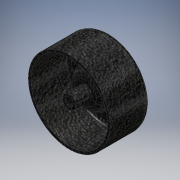
# Autodesk Inventor part: kolo
Saved by Autodesk Inventor 2018 (Build 220112000, 112)
## iProperties
Created: 2023-12-05
Part Number: kolo
Material: Všeobecné
Document SubType Name: Modeling
Designer: 42073
Density: 1 g/cm^3
Appearance: Černý – litý
Author: 42073
Autodesk Inventor part; units mm, degrees
ref_plane "YZ Plane" through (0, 0, 0) normal (1, 0, 0) x (0, 1, 0)
ref_plane "XY Plane" through (0, 0, 0) normal (0, 0, 1) x (1, 0, 0)
sketch "Náčrt1" plane through (0, 0, 0) normal (0, 0, 1) x (1, 0, 0)
  line L0 (0, 0) -> (0, 14.75)
  line L1 (0, 0) -> (15, 0)
  line L2 (15, 0) -> (15, 7)
  line L3 (15, 7) -> (9, 7)
  line L4 (9, 7) -> (9, 14.75)
  arc A0 (9, 14.75) -> (0, 14.75) centre (4.5, -25.625) ccw
  dimension "d1" = 15
  dimension "d2" = 7
  dimension "d3" = 6
  constraints: 10 end point, 3 perpendicular, 2 point on circle, 1 centre point, 1 horizontal, 1 vertical
  measures "d1" distance of L0.start L1.end
  measures "d2" distance of L1.end L2.end
  measures "d3" distance of L2.end L3.end
revolve "Rotace1" add sketch "Náčrt1" angle 360 about axis through (15, 0, 0) along (0, 1, 0)
sketch "Náčrt2" plane through (15, 0, 0) normal (0, -1, 0) x (1, 0, 0)
  circle A0 centre (0, 0) radius 1.5
  point P0 (-15, 0)
  dimension "d6" = 3
  constraints: 1 centre point
  measures "d6" diameter of A0
extrude "Vysunutí1" cut sketch "Náčrt2" against normal blind 10
fillet "Zaoblení1" radius 2 3 edges at (21, 7, 0) (21, 14.75, 0) (30, 14.75, 0)
shell "Skořepina1" thickness 1 removed faces 1 at (4.6453, 0, -1.1966)
ref_plane "Pracovní rovina1" through (0, 15.25, 0) normal (0, 1, 0) x (-1, 0, 0)
sketch "Náčrt3" plane through (0, 15.25, 0) normal (0, 1, 0) x (-1, 0, 0)
  circle A0 centre (-15, 0) radius 1.5 projected
  circle A1 centre (-15, 0) radius 9.5
  line L0 (-24.5881, -0.0196) -> (-27.472, 1.4048)
  line L1 (-27.472, 1.4048) -> (-27.4055, 1.8993)
  line L2 (-27.4055, 1.8993) -> (-24.2478, 2.5116)
  line L3 (-24.2478, 2.5116) -> (-24.3048, 2.0881)
  line L4 (-24.3048, 2.0881) -> (-25.1862, 1.9275)
  line L5 (-25.1862, 1.9275) -> (-25.3412, 0.7745)
  line L6 (-25.3412, 0.7745) -> (-24.5335, 0.3868)
  line L7 (-24.5335, 0.3868) -> (-24.5881, -0.0196)
  line L8 (-25.5437, 1.8634) -> (-27.0288, 1.587)
  line L9 (-27.0288, 1.587) -> (-25.6691, 0.9307)
  line L10 (-25.6691, 0.9307) -> (-25.5437, 1.8634)
  line L11 (-23.4586, 4.4131) -> (-23.6046, 4.0565)
  line L12 (-23.6046, 4.0565) -> (-23.8195, 4.1445)
  spline S0 degree 2 poles (-23.8195, 4.1445) (-23.7846, 4.0341) (-23.7427, 3.8755) (-23.7376, 3.7773) knots 0 0 0 1 2 2 2
  spline S1 degree 2 poles (-23.7376, 3.7773) (-23.7319, 3.6869) (-23.7595, 3.5087) (-23.8034, 3.4013) knots 0 0 0 1 2 2 2
  spline S2 degree 2 poles (-23.8034, 3.4013) (-23.8746, 3.2275) (-24.1384, 2.9939) (-24.3199, 2.9481) knots 0 0 0 1 2 2 2
  spline S3 degree 2 poles (-24.3199, 2.9481) (-24.5015, 2.9023) (-24.9597, 2.9565) (-25.2272, 3.066) knots 0 0 0 1 2 2 2
  spline S4 degree 2 poles (-25.2272, 3.066) (-25.506, 3.1802) (-25.854, 3.4908) (-25.9556, 3.6792) knots 0 0 0 1 2 2 2
  spline S5 degree 2 poles (-25.9556, 3.6792) (-26.0451, 3.8519) (-26.069, 4.2434) (-25.995, 4.4239) knots 0 0 0 1 2 2 2
  spline S6 degree 2 poles (-25.995, 4.4239) (-25.9305, 4.5817) (-25.7632, 4.7881) (-25.6367, 4.8885) knots 0 0 0 1 2 2 2
  line L13 (-25.6367, 4.8885) -> (-26.5511, 5.2628)
  line L14 (-26.5511, 5.2628) -> (-26.4051, 5.6194)
  line L15 (-26.4051, 5.6194) -> (-23.4586, 4.4131)
  line L16 (-24.1189, 4.2671) -> (-25.3418, 4.7677)
  spline S7 degree 2 poles (-25.3418, 4.7677) (-25.4601, 4.6614) (-25.5942, 4.4707) (-25.6438, 4.3496) knots 0 0 0 1 2 2 2
  spline S8 degree 2 poles (-25.6438, 4.3496) (-25.7561, 4.0752) (-25.4719, 3.5959) (-25.0833, 3.4368) knots 0 0 0 1 2 2 2
  spline S9 degree 2 poles (-25.0833, 3.4368) (-24.7085, 3.2834) (-24.2157, 3.3592) (-24.1081, 3.6221) knots 0 0 0 1 2 2 2
  spline S10 degree 2 poles (-24.1081, 3.6221) (-24.051, 3.7615) (-24.0629, 4.0974) (-24.1189, 4.2671) knots 0 0 0 1 2 2 2
  spline S11 degree 2 poles (-22.5603, 5.669) (-22.8813, 5.2245) (-23.7328, 5.096) (-24.1933, 5.4287) knots 0 0 0 1 2 2 2
  spline S12 degree 2 poles (-24.1933, 5.4287) (-24.6459, 5.7555) (-24.8398, 6.6176) (-24.5635, 7.0001) knots 0 0 0 1 2 2 2
  spline S13 degree 2 poles (-24.5635, 7.0001) (-24.4392, 7.1723) (-24.1467, 7.3663) (-23.9697, 7.3878) knots 0 0 0 1 2 2 2
  spline S14 degree 2 poles (-23.9697, 7.3878) (-23.7913, 7.4112) (-23.4083, 7.2961) (-23.186, 7.1356) knots 0 0 0 1 2 2 2
  line L17 (-23.186, 7.1356) -> (-23.0158, 7.0127)
  line L18 (-23.0158, 7.0127) -> (-23.9428, 5.7291)
  spline S15 degree 2 poles (-23.9428, 5.7291) (-23.6204, 5.4963) (-23.0437, 5.5734) (-22.8355, 5.8617) knots 0 0 0 1 2 2 2
  spline S16 degree 2 poles (-22.8355, 5.8617) (-22.7617, 5.9638) (-22.6646, 6.1953) (-22.6428, 6.3015) knots 0 0 0 1 2 2 2
  spline S17 degree 2 poles (-22.6428, 6.3015) (-22.6221, 6.4145) (-22.6083, 6.5812) (-22.6129, 6.6424) knots 0 0 0 1 2 2 2
  line L19 (-22.6129, 6.6424) -> (-22.5999, 6.6604)
  line L20 (-22.5999, 6.6604) -> (-22.2595, 6.4146)
  spline S18 degree 2 poles (-22.2595, 6.4146) (-22.2765, 6.3446) (-22.331, 6.1342) (-22.3593, 6.0571) knots 0 0 0 1 2 2 2
  spline S19 degree 2 poles (-22.3593, 6.0571) (-22.3983, 5.9482) (-22.4793, 5.7812) (-22.5603, 5.669) knots 0 0 0 1 2 2 2
  spline S20 degree 2 poles (-23.4739, 6.8804) (-23.6029, 6.9675) (-23.8248, 7.0485) (-23.923, 7.0433) knots 0 0 0 1 2 2 2
  spline S21 degree 2 poles (-23.923, 7.0433) (-24.0321, 7.0398) (-24.2291, 6.9231) (-24.3203, 6.797) knots 0 0 0 1 2 2 2
  spline S22 degree 2 poles (-24.3203, 6.797) (-24.4099, 6.6728) (-24.4616, 6.4451) (-24.4416, 6.321) knots 0 0 0 1 2 2 2
  spline S23 degree 2 poles (-24.4416, 6.321) (-24.4182, 6.1974) (-24.292, 5.9966) (-24.1811, 5.9012) knots 0 0 0 1 2 2 2
  line L21 (-24.1811, 5.9012) -> (-23.4739, 6.8804)
  spline S24 degree 2 poles (-21.1682, 8.734) (-20.7912, 8.2959) (-20.8017, 7.456) (-21.1536, 7.1531) knots 0 0 0 1 2 2 2
  spline S25 degree 2 poles (-21.1536, 7.1531) (-21.515, 6.8421) (-22.3525, 6.9785) (-22.7166, 7.4016) knots 0 0 0 1 2 2 2
  spline S26 degree 2 poles (-22.7166, 7.4016) (-23.0904, 7.836) (-23.0775, 8.6845) (-22.7293, 8.9841) knots 0 0 0 1 2 2 2
  spline S27 degree 2 poles (-22.7293, 8.9841) (-22.3773, 9.287) (-21.5436, 9.1702) (-21.1682, 8.734) knots 0 0 0 1 2 2 2
  spline S28 degree 2 poles (-21.4697, 8.4746) (-21.7597, 8.8116) (-22.2869, 8.9282) (-22.5134, 8.7333) knots 0 0 0 1 2 2 2
  spline S29 degree 2 poles (-22.5134, 8.7333) (-22.74, 8.5383) (-22.7052, 7.998) (-22.4152, 7.661) knots 0 0 0 1 2 2 2
  spline S30 degree 2 poles (-22.4152, 7.661) (-22.1332, 7.3334) (-21.5961, 7.209) (-21.3695, 7.404) knots 0 0 0 1 2 2 2
  spline S31 degree 2 poles (-21.3695, 7.404) (-21.1449, 7.5973) (-21.1829, 8.1413) (-21.4697, 8.4746) knots 0 0 0 1 2 2 2
  line L22 (-18.4856, 8.8838) -> (-18.8293, 8.7096)
  line L23 (-18.8293, 8.7096) -> (-19.4189, 9.873)
  spline S32 degree 2 poles (-19.4189, 9.873) (-19.4903, 10.014) (-19.6396, 10.2429) (-19.7161, 10.2955) knots 0 0 0 1 2 2 2
  spline S33 degree 2 poles (-19.7161, 10.2955) (-19.797, 10.3514) (-19.9848, 10.3504) (-20.1126, 10.2857) knots 0 0 0 1 2 2 2
  spline S34 degree 2 poles (-20.1126, 10.2857) (-20.2404, 10.2209) (-20.4421, 9.947) (-20.5163, 9.771) knots 0 0 0 1 2 2 2
  line L24 (-20.5163, 9.771) -> (-19.7437, 8.2463)
  line L25 (-19.7437, 8.2463) -> (-20.0874, 8.0721)
  line L26 (-20.0874, 8.0721) -> (-21.1213, 10.1123)
  line L27 (-21.1213, 10.1123) -> (-20.7776, 10.2865)
  line L28 (-20.7776, 10.2865) -> (-20.6626, 10.0596)
  spline S35 degree 2 poles (-20.6626, 10.0596) (-20.5787, 10.2765) (-20.3549, 10.5727) (-20.1875, 10.6575) knots 0 0 0 1 2 2 2
  spline S36 degree 2 poles (-20.1875, 10.6575) (-19.8878, 10.8094) (-19.3476, 10.5847) (-19.1566, 10.208) knots 0 0 0 1 2 2 2
  line L29 (-19.1566, 10.208) -> (-18.4856, 8.8838)
  line L30 (-15.1164, 12.231) -> (-16.5279, 12.0972)
  line L31 (-16.5279, 12.0972) -> (-16.4467, 11.2414)
  line L32 (-16.4467, 11.2414) -> (-15.0943, 11.3697)
  line L33 (-15.0943, 11.3697) -> (-15.0603, 11.0107)
  line L34 (-15.0603, 11.0107) -> (-16.4127, 10.8824)
  line L35 (-16.4127, 10.8824) -> (-16.2742, 9.4218)
  line L36 (-16.2742, 9.4218) -> (-16.6775, 9.3836)
  line L37 (-16.6775, 9.3836) -> (-16.9652, 12.4179)
  line L38 (-16.9652, 12.4179) -> (-15.1505, 12.59)
  line L39 (-15.1505, 12.59) -> (-15.1164, 12.231)
  line L40 (-12.8787, 9.2951) -> (-14.3511, 9.5023)
  line L41 (-14.3511, 9.5023) -> (-14.3078, 9.8105)
  line L42 (-14.3078, 9.8105) -> (-13.7599, 9.7334)
  line L43 (-13.7599, 9.7334) -> (-13.4752, 11.7562)
  line L44 (-13.4752, 11.7562) -> (-14.0231, 11.8333)
  line L45 (-14.0231, 11.8333) -> (-13.9842, 12.1096)
  spline S37 degree 2 poles (-13.9842, 12.1096) (-13.6736, 12.0659) (-13.3553, 12.2007) (-13.3013, 12.4426) knots 0 0 0 1 2 2 2
  line L46 (-13.3013, 12.4426) -> (-12.9882, 12.3985)
  line L47 (-12.9882, 12.3985) -> (-13.371, 9.6786)
  line L48 (-13.371, 9.6786) -> (-12.8353, 9.6033)
  line L49 (-12.8353, 9.6033) -> (-12.8787, 9.2951)
  line L50 (-10.4121, 8.3212) -> (-9.0641, 10.6461)
  line L51 (-9.0641, 10.6461) -> (-9.9487, 11.159)
  line L52 (-9.9487, 11.159) -> (-9.7678, 11.471)
  line L53 (-9.7678, 11.471) -> (-7.6481, 10.2419)
  line L54 (-7.6481, 10.2419) -> (-7.829, 9.9299)
  line L55 (-7.829, 9.9299) -> (-8.7136, 10.4429)
  line L56 (-8.7136, 10.4429) -> (-10.0616, 8.118)
  line L57 (-10.0616, 8.118) -> (-10.4121, 8.3212)
  spline S38 degree 2 poles (-8.3061, 6.6699) (-8.7001, 7.0514) (-8.7052, 7.9125) (-8.31, 8.3206) knots 0 0 0 1 2 2 2
  spline S39 degree 2 poles (-8.31, 8.3206) (-7.9217, 8.7216) (-7.0407, 8.79) (-6.7018, 8.4618) knots 0 0 0 1 2 2 2
  spline S40 degree 2 poles (-6.7018, 8.4618) (-6.5492, 8.314) (-6.3991, 7.9968) (-6.4032, 7.8185) knots 0 0 0 1 2 2 2
  spline S41 degree 2 poles (-6.4032, 7.8185) (-6.4055, 7.6386) (-6.5744, 7.276) (-6.7651, 7.0791) knots 0 0 0 1 2 2 2
  line L58 (-6.7651, 7.0791) -> (-6.9111, 6.9282)
  line L59 (-6.9111, 6.9282) -> (-8.0486, 8.0296)
  spline S42 degree 2 poles (-8.0486, 8.0296) (-8.3252, 7.7439) (-8.3315, 7.1621) (-8.076, 6.9147) knots 0 0 0 1 2 2 2
  spline S43 degree 2 poles (-8.076, 6.9147) (-7.9855, 6.8271) (-7.7703, 6.6978) (-7.6684, 6.661) knots 0 0 0 1 2 2 2
  spline S44 degree 2 poles (-7.6684, 6.661) (-7.5595, 6.6243) (-7.3965, 6.5868) (-7.3353, 6.5825) knots 0 0 0 1 2 2 2
  line L60 (-7.3353, 6.5825) -> (-7.3193, 6.5671)
  line L61 (-7.3193, 6.5671) -> (-7.6114, 6.2654)
  spline S45 degree 2 poles (-7.6114, 6.2654) (-7.6782, 6.2923) (-7.8787, 6.3764) (-7.9509, 6.4154) knots 0 0 0 1 2 2 2
  spline S46 degree 2 poles (-7.9509, 6.4154) (-8.0531, 6.4696) (-8.2068, 6.5737) (-8.3061, 6.6699) knots 0 0 0 1 2 2 2
  spline S47 degree 2 poles (-6.9764, 7.4006) (-6.8717, 7.5158) (-6.7597, 7.7237) (-6.7508, 7.8217) knots 0 0 0 1 2 2 2
  spline S48 degree 2 poles (-6.7508, 7.8217) (-6.7386, 7.9302) (-6.8259, 8.1419) (-6.9377, 8.2501) knots 0 0 0 1 2 2 2
  spline S49 degree 2 poles (-6.9377, 8.2501) (-7.0477, 8.3567) (-7.2656, 8.4405) (-7.3914, 8.4385) knots 0 0 0 1 2 2 2
  spline S50 degree 2 poles (-7.3914, 8.4385) (-7.5171, 8.4329) (-7.7339, 8.3369) (-7.8441, 8.2408) knots 0 0 0 1 2 2 2
  line L62 (-7.8441, 8.2408) -> (-6.9764, 7.4006)
  spline S51 degree 2 poles (-6.5566, 4.8808) (-6.6111, 4.9016) (-6.8004, 4.9679) (-6.8716, 5.0103) knots 0 0 0 1 2 2 2
  spline S52 degree 2 poles (-6.8716, 5.0103) (-6.972, 5.0662) (-7.1226, 5.1955) (-7.216, 5.341) knots 0 0 0 1 2 2 2
  spline S53 degree 2 poles (-7.216, 5.341) (-7.292, 5.4595) (-7.34, 5.731) (-7.311, 5.8641) knots 0 0 0 1 2 2 2
  spline S54 degree 2 poles (-7.311, 5.8641) (-7.2814, 5.9917) (-7.1086, 6.2347) (-6.9797, 6.3174) knots 0 0 0 1 2 2 2
  spline S55 degree 2 poles (-6.9797, 6.3174) (-6.7802, 6.4455) (-6.3894, 6.4586) (-6.1909, 6.3277) knots 0 0 0 1 2 2 2
  spline S56 degree 2 poles (-6.1909, 6.3277) (-6.012, 6.2136) (-5.6731, 5.8089) (-5.4944, 5.5626) knots 0 0 0 1 2 2 2
  line L63 (-5.4944, 5.5626) -> (-5.432, 5.6026)
  spline S57 degree 2 poles (-5.432, 5.6026) (-5.3198, 5.6746) (-5.2245, 5.8326) (-5.2251, 5.9203) knots 0 0 0 1 2 2 2
  spline S58 degree 2 poles (-5.2251, 5.9203) (-5.2256, 6.0081) (-5.3154, 6.2028) (-5.3768, 6.2985) knots 0 0 0 1 2 2 2
  spline S59 degree 2 poles (-5.3768, 6.2985) (-5.4488, 6.4107) (-5.7101, 6.6715) (-5.872, 6.7819) knots 0 0 0 1 2 2 2
  line L64 (-5.872, 6.7819) -> (-5.884, 6.8006)
  line L65 (-5.884, 6.8006) -> (-5.5535, 7.0127)
  spline S60 degree 2 poles (-5.5535, 7.0127) (-5.4712, 6.9393) (-5.194, 6.6447) (-5.0886, 6.4805) knots 0 0 0 1 2 2 2
  spline S61 degree 2 poles (-5.0886, 6.4805) (-4.9605, 6.2809) (-4.8481, 5.9686) (-4.8598, 5.8085) knots 0 0 0 1 2 2 2
  spline S62 degree 2 poles (-4.8598, 5.8085) (-4.8707, 5.6518) (-5.0555, 5.3864) (-5.2364, 5.2703) knots 0 0 0 1 2 2 2
  line L66 (-5.2364, 5.2703) -> (-6.5522, 4.4258)
  line L67 (-6.5522, 4.4258) -> (-6.7603, 4.7501)
  line L68 (-6.7603, 4.7501) -> (-6.5566, 4.8808)
  line L69 (-6.2864, 5.0542) -> (-5.7522, 5.3971)
  spline S63 degree 2 poles (-5.7522, 5.3971) (-5.8373, 5.5069) (-6.0981, 5.8355) (-6.2021, 5.9243) knots 0 0 0 1 2 2 2
  spline S64 degree 2 poles (-6.2021, 5.9243) (-6.3243, 6.0278) (-6.5966, 6.0908) (-6.7421, 5.9974) knots 0 0 0 1 2 2 2
  spline S65 degree 2 poles (-6.7421, 5.9974) (-6.9084, 5.8907) (-6.9566, 5.5955) (-6.8419, 5.4168) knots 0 0 0 1 2 2 2
  spline S66 degree 2 poles (-6.8419, 5.4168) (-6.7445, 5.265) (-6.4535, 5.0996) (-6.2864, 5.0542) knots 0 0 0 1 2 2 2
  line L70 (-5.5505, 1.4817) -> (-4.2753, 1.8375)
  spline S67 degree 2 poles (-4.2753, 1.8375) (-4.123, 1.88) (-3.8704, 1.9762) (-3.8096, 2.0341) knots 0 0 0 1 2 2 2
  spline S68 degree 2 poles (-3.8096, 2.0341) (-3.7417, 2.0941) (-3.7061, 2.2605) (-3.7413, 2.3866) knots 0 0 0 1 2 2 2
  spline S69 degree 2 poles (-3.7413, 2.3866) (-3.7731, 2.5008) (-3.9865, 2.7233) (-4.1583, 2.8241) knots 0 0 0 1 2 2 2
  spline S70 degree 2 poles (-4.1583, 2.8241) (-4.1909, 2.8125) (-4.2824, 2.7818) (-4.3442, 2.7645) knots 0 0 0 1 2 2 2
  line L71 (-4.3442, 2.7645) -> (-5.7955, 2.3596)
  line L72 (-5.7955, 2.3596) -> (-5.8991, 2.7307)
  line L73 (-5.8991, 2.7307) -> (-4.6239, 3.0866)
  spline S71 degree 2 poles (-4.6239, 3.0866) (-4.4716, 3.129) (-4.2189, 3.2252) (-4.1582, 3.2832) knots 0 0 0 1 2 2 2
  spline S72 degree 2 poles (-4.1582, 3.2832) (-4.0903, 3.3432) (-4.0546, 3.5095) (-4.0898, 3.6356) knots 0 0 0 1 2 2 2
  spline S73 degree 2 poles (-4.0898, 3.6356) (-4.123, 3.7546) (-4.3466, 3.9768) (-4.4977, 4.068) knots 0 0 0 1 2 2 2
  line L74 (-4.4977, 4.068) -> (-6.144, 3.6086)
  line L75 (-6.144, 3.6086) -> (-6.2476, 3.9797)
  line L76 (-6.2476, 3.9797) -> (-4.0445, 4.5945)
  line L77 (-4.0445, 4.5945) -> (-3.941, 4.2234)
  line L78 (-3.941, 4.2234) -> (-4.1836, 4.1557)
  spline S74 degree 2 poles (-4.1836, 4.1557) (-3.998, 4.051) (-3.759, 3.81) (-3.7112, 3.6387) knots 0 0 0 1 2 2 2
  spline S75 degree 2 poles (-3.7112, 3.6387) (-3.6567, 3.4436) (-3.7508, 3.0917) (-3.9311, 2.9567) knots 0 0 0 1 2 2 2
  spline S76 degree 2 poles (-3.9311, 2.9567) (-3.6961, 2.8403) (-3.4144, 2.5753) (-3.3626, 2.3897) knots 0 0 0 1 2 2 2
  spline S77 degree 2 poles (-3.3626, 2.3897) (-3.3228, 2.2469) (-3.3457, 1.9892) (-3.4218, 1.8757) knots 0 0 0 1 2 2 2
  spline S78 degree 2 poles (-3.4218, 1.8757) (-3.4971, 1.7598) (-3.7697, 1.5786) (-3.9957, 1.5155) knots 0 0 0 1 2 2 2
  line L79 (-3.9957, 1.5155) -> (-5.4469, 1.1105)
  line L80 (-5.4469, 1.1105) -> (-5.5505, 1.4817)
  line L81 (-4.5134, -1.9382) -> (-4.3655, -0.7942)
  line L82 (-4.3655, -0.7942) -> (-3.9981, -0.8417)
  line L83 (-3.9981, -0.8417) -> (-4.1459, -1.9857)
  line L84 (-4.1459, -1.9857) -> (-4.5134, -1.9382)
  line L85 (-7.2165, -5.6157) -> (-6.9726, -5.1496)
  line L86 (-6.9726, -5.1496) -> (-5.4514, -4.8583)
  line L87 (-5.4514, -4.8583) -> (-5.2361, -4.4469)
  line L88 (-5.2361, -4.4469) -> (-6.3107, -3.8846)
  line L89 (-6.3107, -3.8846) -> (-6.1229, -3.5257)
  line L90 (-6.1229, -3.5257) -> (-3.4223, -4.9388)
  line L91 (-3.4223, -4.9388) -> (-3.7864, -5.6347)
  spline S79 degree 2 poles (-3.7864, -5.6347) (-3.9078, -5.8667) (-4.1219, -6.1534) (-4.2882, -6.2475) knots 0 0 0 1 2 2 2
  spline S80 degree 2 poles (-4.2882, -6.2475) (-4.4546, -6.3417) (-4.8272, -6.3558) (-5.0395, -6.2447) knots 0 0 0 1 2 2 2
  spline S81 degree 2 poles (-5.0395, -6.2447) (-5.3349, -6.0901) (-5.5774, -5.5785) (-5.5386, -5.2699) knots 0 0 0 1 2 2 2
  line L92 (-5.5386, -5.2699) -> (-7.2165, -5.6157)
  spline S82 degree 2 poles (-4.8721, -5.8556) (-4.7539, -5.9174) (-4.5288, -5.9293) (-4.4239, -5.8727) knots 0 0 0 1 2 2 2
  spline S83 degree 2 poles (-4.4239, -5.8727) (-4.3334, -5.8224) (-4.1854, -5.6407) (-4.1075, -5.4918) knots 0 0 0 1 2 2 2
  line L93 (-4.1075, -5.4918) -> (-3.9208, -5.1351)
  line L94 (-3.9208, -5.1351) -> (-4.9363, -4.6038)
  line L95 (-4.9363, -4.6038) -> (-5.1012, -4.9189)
  spline S84 degree 2 poles (-5.1012, -4.9189) (-5.1825, -5.0743) (-5.2572, -5.3502) (-5.2165, -5.4802) knots 0 0 0 1 2 2 2
  spline S85 degree 2 poles (-5.2165, -5.4802) (-5.1833, -5.598) (-5.0122, -5.7823) (-4.8721, -5.8556) knots 0 0 0 1 2 2 2
  spline S86 degree 2 poles (-8.0663, -6.8583) (-8.0605, -6.8003) (-8.0465, -6.6002) (-8.0244, -6.5203) knots 0 0 0 1 2 2 2
  spline S87 degree 2 poles (-8.0244, -6.5203) (-7.9969, -6.4087) (-7.9118, -6.2294) (-7.7961, -6.101) knots 0 0 0 1 2 2 2
  spline S88 degree 2 poles (-7.7961, -6.101) (-7.7018, -5.9964) (-7.4526, -5.8785) (-7.3166, -5.8714) knots 0 0 0 1 2 2 2
  spline S89 degree 2 poles (-7.3166, -5.8714) (-7.1857, -5.8663) (-6.9057, -5.969) (-6.792, -6.0715) knots 0 0 0 1 2 2 2
  spline S90 degree 2 poles (-6.792, -6.0715) (-6.6158, -6.2302) (-6.5002, -6.6037) (-6.5742, -6.8297) knots 0 0 0 1 2 2 2
  spline S91 degree 2 poles (-6.5742, -6.8297) (-6.6371, -7.0323) (-6.9381, -7.466) (-7.1286, -7.7032) knots 0 0 0 1 2 2 2
  line L96 (-7.1286, -7.7032) -> (-7.0736, -7.7528)
  spline S92 degree 2 poles (-7.0736, -7.7528) (-6.9745, -7.8421) (-6.797, -7.8924) (-6.7125, -7.8687) knots 0 0 0 1 2 2 2
  spline S93 degree 2 poles (-6.7125, -7.8687) (-6.628, -7.8451) (-6.4638, -7.7071) (-6.3878, -7.6227) knots 0 0 0 1 2 2 2
  spline S94 degree 2 poles (-6.3878, -7.6227) (-6.2985, -7.5237) (-6.1158, -7.2028) (-6.052, -7.0176) knots 0 0 0 1 2 2 2
  line L97 (-6.052, -7.0176) -> (-6.0371, -7.0011)
  line L98 (-6.0371, -7.0011) -> (-5.7453, -7.264)
  spline S95 degree 2 poles (-5.7453, -7.264) (-5.7944, -7.3628) (-6.0056, -7.7078) (-6.1362, -7.8528) knots 0 0 0 1 2 2 2
  spline S96 degree 2 poles (-6.1362, -7.8528) (-6.2949, -8.0289) (-6.5666, -8.2197) (-6.7241, -8.2506) knots 0 0 0 1 2 2 2
  spline S97 degree 2 poles (-6.7241, -8.2506) (-6.8782, -8.2814) (-7.1829, -8.173) (-7.3425, -8.0292) knots 0 0 0 1 2 2 2
  line L99 (-7.3425, -8.0292) -> (-8.504, -6.9825)
  line L100 (-8.504, -6.9825) -> (-8.2461, -6.6963)
  line L101 (-8.2461, -6.6963) -> (-8.0663, -6.8583)
  line L102 (-7.8277, -7.0733) -> (-7.3561, -7.4982)
  spline S98 degree 2 poles (-7.3561, -7.4982) (-7.2727, -7.3872) (-7.0245, -7.049) (-6.9662, -6.9253) knots 0 0 0 1 2 2 2
  spline S99 degree 2 poles (-6.9662, -6.9253) (-6.8985, -6.7801) (-6.9096, -6.5008) (-7.038, -6.3851) knots 0 0 0 1 2 2 2
  spline S100 degree 2 poles (-7.038, -6.3851) (-7.1848, -6.2528) (-7.4822, -6.284) (-7.6245, -6.4418) knots 0 0 0 1 2 2 2
  spline S101 degree 2 poles (-7.6245, -6.4418) (-7.7452, -6.5758) (-7.828, -6.9001) (-7.8277, -7.0733) knots 0 0 0 1 2 2 2
  spline S102 degree 2 poles (-9.6855, -7.8149) (-9.4926, -7.677) (-9.0884, -7.5672) (-8.8877, -7.6059) knots 0 0 0 1 2 2 2
  spline S103 degree 2 poles (-8.8877, -7.6059) (-8.6884, -7.6425) (-8.3004, -7.9178) (-8.1251, -8.1629) knots 0 0 0 1 2 2 2
  spline S104 degree 2 poles (-8.1251, -8.1629) (-7.9499, -8.4081) (-7.8248, -8.8591) (-7.8492, -9.0587) knots 0 0 0 1 2 2 2
  spline S105 degree 2 poles (-7.8492, -9.0587) (-7.8721, -9.2603) (-8.1062, -9.625) (-8.2951, -9.76) knots 0 0 0 1 2 2 2
  spline S106 degree 2 poles (-8.2951, -9.76) (-8.4478, -9.8692) (-8.7949, -9.9867) (-8.9457, -10.0095) knots 0 0 0 1 2 2 2
  line L103 (-8.9457, -10.0095) -> (-9.197, -9.6578)
  line L104 (-9.197, -9.6578) -> (-9.179, -9.6449)
  spline S107 degree 2 poles (-9.179, -9.6449) (-9.1247, -9.6486) (-8.9685, -9.6463) (-8.8668, -9.6313) knots 0 0 0 1 2 2 2
  spline S108 degree 2 poles (-8.8668, -9.6313) (-8.7776, -9.616) (-8.5648, -9.5399) (-8.4844, -9.4824) knots 0 0 0 1 2 2 2
  spline S109 degree 2 poles (-8.4844, -9.4824) (-8.2413, -9.3086) (-8.2088, -8.7297) (-8.4486, -8.3942) knots 0 0 0 1 2 2 2
  spline S110 degree 2 poles (-8.4486, -8.3942) (-8.6828, -8.0666) (-9.231, -7.9029) (-9.4842, -8.0839) knots 0 0 0 1 2 2 2
  spline S111 degree 2 poles (-9.4842, -8.0839) (-9.6369, -8.193) (-9.8237, -8.5178) (-9.8598, -8.6924) knots 0 0 0 1 2 2 2
  line L105 (-9.8598, -8.6924) -> (-9.8779, -8.7054)
  line L106 (-9.8779, -8.7054) -> (-10.1292, -8.3537)
  spline S112 degree 2 poles (-10.1292, -8.3537) (-10.0988, -8.2986) (-10.0027, -8.1357) (-9.9565, -8.0814) knots 0 0 0 1 2 2 2
  spline S113 degree 2 poles (-9.9565, -8.0814) (-9.8933, -7.9999) (-9.784, -7.8853) (-9.6855, -7.8149) knots 0 0 0 1 2 2 2
  line L107 (-10.8799, -8.5623) -> (-10.5362, -8.3882)
  line L108 (-10.5362, -8.3882) -> (-9.5029, -10.4287)
  line L109 (-9.5029, -10.4287) -> (-9.8466, -10.6028)
  line L110 (-9.8466, -10.6028) -> (-10.8799, -8.5623)
  line L111 (-9.699, -10.9544) -> (-9.309, -10.7569)
  line L112 (-9.309, -10.7569) -> (-9.1282, -11.1139)
  line L113 (-9.1282, -11.1139) -> (-9.5182, -11.3114)
  line L114 (-9.5182, -11.3114) -> (-9.699, -10.9544)
  line L115 (-13.096, -9.3513) -> (-12.7274, -9.2389)
  line L116 (-12.7274, -9.2389) -> (-12.347, -10.4863)
  spline S114 degree 2 poles (-12.347, -10.4863) (-12.3009, -10.6375) (-12.1933, -10.8888) (-12.127, -10.9538) knots 0 0 0 1 2 2 2
  spline S115 degree 2 poles (-12.127, -10.9538) (-12.0569, -11.0228) (-11.8717, -11.0541) (-11.7347, -11.0123) knots 0 0 0 1 2 2 2
  spline S116 degree 2 poles (-11.7347, -11.0123) (-11.5976, -10.9705) (-11.3517, -10.7354) (-11.2484, -10.5748) knots 0 0 0 1 2 2 2
  line L117 (-11.2484, -10.5748) -> (-11.7469, -8.9399)
  line L118 (-11.7469, -8.9399) -> (-11.3784, -8.8275)
  line L119 (-11.3784, -8.8275) -> (-10.7112, -11.0152)
  line L120 (-10.7112, -11.0152) -> (-11.0798, -11.1276)
  line L121 (-11.0798, -11.1276) -> (-11.154, -10.8843)
  spline S117 degree 2 poles (-11.154, -10.8843) (-11.274, -11.0836) (-11.5454, -11.3368) (-11.7249, -11.3915) knots 0 0 0 1 2 2 2
  spline S118 degree 2 poles (-11.7249, -11.3915) (-12.0462, -11.4895) (-12.5398, -11.1752) (-12.663, -10.7712) knots 0 0 0 1 2 2 2
  line L122 (-12.663, -10.7712) -> (-13.096, -9.3513)
  spline S119 degree 2 poles (-13.7259, -9.0803) (-13.7662, -9.0651) (-13.9195, -9.0187) (-14.0169, -9.0015) knots 0 0 0 1 2 2 2
  spline S120 degree 2 poles (-14.0169, -9.0015) (-14.1244, -8.9799) (-14.3061, -8.9573) (-14.4122, -8.9628) knots 0 0 0 1 2 2 2
  spline S121 degree 2 poles (-14.4122, -8.9628) (-14.5898, -8.9721) (-14.8315, -9.0788) (-14.8962, -9.1662) knots 0 0 0 1 2 2 2
  spline S122 degree 2 poles (-14.8962, -9.1662) (-14.9584, -9.2536) (-14.9987, -9.4758) (-14.9914, -9.6164) knots 0 0 0 1 2 2 2
  line L123 (-14.9914, -9.6164) -> (-14.9809, -9.8162)
  spline S123 degree 2 poles (-14.9809, -9.8162) (-14.8326, -9.6724) (-14.5409, -9.5285) (-14.3164, -9.5168) knots 0 0 0 1 2 2 2
  spline S124 degree 2 poles (-14.3164, -9.5168) (-13.9267, -9.4964) (-13.4351, -10.0519) (-13.4065, -10.597) knots 0 0 0 1 2 2 2
  spline S125 degree 2 poles (-13.4065, -10.597) (-13.3917, -10.8807) (-13.5291, -11.3282) (-13.6541, -11.4905) knots 0 0 0 1 2 2 2
  spline S126 degree 2 poles (-13.6541, -11.4905) (-13.7748, -11.6428) (-14.1191, -11.8216) (-14.3066, -11.8314) knots 0 0 0 1 2 2 2
  spline S127 degree 2 poles (-14.3066, -11.8314) (-14.4842, -11.8407) (-14.7476, -11.7704) (-14.8823, -11.7007) knots 0 0 0 1 2 2 2
  line L124 (-14.8823, -11.7007) -> (-14.8995, -11.7981)
  line L125 (-14.8995, -11.7981) -> (-15.2621, -11.8171)
  line L126 (-15.2621, -11.8171) -> (-15.3679, -9.7944)
  spline S128 degree 2 poles (-15.3679, -9.7944) (-15.3984, -9.2123) (-14.9211, -8.6432) (-14.4007, -8.6159) knots 0 0 0 1 2 2 2
  spline S129 degree 2 poles (-14.4007, -8.6159) (-14.2329, -8.6072) (-13.8798, -8.6431) (-13.727, -8.6796) knots 0 0 0 1 2 2 2
  line L127 (-13.727, -8.6796) -> (-13.7061, -9.0792)
  line L128 (-13.7061, -9.0792) -> (-13.7259, -9.0803)
  line L129 (-14.9644, -10.132) -> (-14.8987, -11.3875)
  spline S130 degree 2 poles (-14.8987, -11.3875) (-14.752, -11.4491) (-14.5072, -11.4956) (-14.3863, -11.4893) knots 0 0 0 1 2 2 2
  spline S131 degree 2 poles (-14.3863, -11.4893) (-14.0952, -11.474) (-13.7822, -11.0273) (-13.8033, -10.6252) knots 0 0 0 1 2 2 2
  spline S132 degree 2 poles (-13.8033, -10.6252) (-13.8232, -10.2454) (-14.098, -9.8615) (-14.3842, -9.8765) knots 0 0 0 1 2 2 2
  spline S133 degree 2 poles (-14.3842, -9.8765) (-14.5346, -9.8844) (-14.8441, -10.0193) (-14.9644, -10.132) knots 0 0 0 1 2 2 2
  line L130 (-21.609, -10.8232) -> (-19.7093, -8.3196)
  line L131 (-19.7093, -8.3196) -> (-19.2913, -8.4978)
  line L132 (-19.2913, -8.4978) -> (-19.7128, -11.0677)
  line L133 (-19.7128, -11.0677) -> (-18.1665, -8.9773)
  line L134 (-18.1665, -8.9773) -> (-17.753, -9.1536)
  line L135 (-17.753, -9.1536) -> (-18.2326, -12.2626)
  line L136 (-18.2326, -12.2626) -> (-18.6166, -12.0989)
  line L137 (-18.6166, -12.0989) -> (-18.1891, -9.5342)
  line L138 (-18.1891, -9.5342) -> (-19.739, -11.6204)
  line L139 (-19.739, -11.6204) -> (-20.1185, -11.4586)
  line L140 (-20.1185, -11.4586) -> (-19.6794, -8.8667)
  line L141 (-19.6794, -8.8667) -> (-21.2432, -10.9791)
  line L142 (-21.2432, -10.9791) -> (-21.609, -10.8232)
  line L143 (-21.9566, -6.5328) -> (-21.6674, -6.7873)
  line L144 (-21.6674, -6.7873) -> (-22.529, -7.7663)
  spline S134 degree 2 poles (-22.529, -7.7663) (-22.6334, -7.885) (-22.7907, -8.1086) (-22.8111, -8.1991) knots 0 0 0 1 2 2 2
  spline S135 degree 2 poles (-22.8111, -8.1991) (-22.833, -8.295) (-22.7624, -8.469) (-22.6549, -8.5637) knots 0 0 0 1 2 2 2
  spline S136 degree 2 poles (-22.6549, -8.5637) (-22.5473, -8.6583) (-22.2181, -8.7441) (-22.0271, -8.7476) knots 0 0 0 1 2 2 2
  line L145 (-22.0271, -8.7476) -> (-20.8979, -7.4645)
  line L146 (-20.8979, -7.4645) -> (-20.6086, -7.7191)
  line L147 (-20.6086, -7.7191) -> (-22.712, -10.1092)
  line L148 (-22.712, -10.1092) -> (-23.0013, -9.8546)
  line L149 (-23.0013, -9.8546) -> (-22.2409, -8.9905)
  spline S137 degree 2 poles (-22.2409, -8.9905) (-22.4735, -8.9931) (-22.8315, -8.8952) (-22.9724, -8.7712) knots 0 0 0 1 2 2 2
  spline S138 degree 2 poles (-22.9724, -8.7712) (-23.2246, -8.5493) (-23.2164, -7.9642) (-22.9374, -7.6471) knots 0 0 0 1 2 2 2
  line L150 (-22.9374, -7.6471) -> (-21.9566, -6.5328)
  spline S139 degree 2 poles (-22.8349, -5.2831) (-22.5202, -5.7321) (-22.6781, -6.5787) (-23.1433, -6.9047) knots 0 0 0 1 2 2 2
  spline S140 degree 2 poles (-23.1433, -6.9047) (-23.6005, -7.225) (-24.4785, -7.1254) (-24.7493, -6.739) knots 0 0 0 1 2 2 2
  spline S141 degree 2 poles (-24.7493, -6.739) (-24.8711, -6.5651) (-24.9585, -6.2252) (-24.9208, -6.0509) knots 0 0 0 1 2 2 2
  spline S142 degree 2 poles (-24.9208, -6.0509) (-24.8844, -5.8747) (-24.65, -5.5506) (-24.4255, -5.3933) knots 0 0 0 1 2 2 2
  line L151 (-24.4255, -5.3933) -> (-24.2535, -5.2728)
  line L152 (-24.2535, -5.2728) -> (-23.345, -6.5694)
  spline S143 degree 2 poles (-23.345, -6.5694) (-23.0193, -6.3413) (-22.903, -5.7712) (-23.1071, -5.4799) knots 0 0 0 1 2 2 2
  spline S144 degree 2 poles (-23.1071, -5.4799) (-23.1794, -5.3767) (-23.3663, -5.209) (-23.4594, -5.1536) knots 0 0 0 1 2 2 2
  spline S145 degree 2 poles (-23.4594, -5.1536) (-23.5594, -5.097) (-23.7124, -5.0293) (-23.7717, -5.0136) knots 0 0 0 1 2 2 2
  line L153 (-23.7717, -5.0136) -> (-23.7844, -4.9954)
  line L154 (-23.7844, -4.9954) -> (-23.4405, -4.7544)
  spline S146 degree 2 poles (-23.4405, -4.7544) (-23.38, -4.7934) (-23.1991, -4.9139) (-23.1355, -4.9659) knots 0 0 0 1 2 2 2
  spline S147 degree 2 poles (-23.1355, -4.9659) (-23.0454, -5.0385) (-22.9142, -5.1698) (-22.8349, -5.2831) knots 0 0 0 1 2 2 2
  spline S148 degree 2 poles (-24.2788, -5.7489) (-24.4034, -5.8423) (-24.5527, -6.0253) (-24.58, -6.1198) knots 0 0 0 1 2 2 2
  spline S149 degree 2 poles (-24.58, -6.1198) (-24.6125, -6.224) (-24.5669, -6.4484) (-24.4776, -6.5758) knots 0 0 0 1 2 2 2
  spline S150 degree 2 poles (-24.4776, -6.5758) (-24.3897, -6.7012) (-24.1915, -6.8248) (-24.0677, -6.8466) knots 0 0 0 1 2 2 2
  spline S151 degree 2 poles (-24.0677, -6.8466) (-23.9432, -6.8649) (-23.7122, -6.8116) (-23.5857, -6.7381) knots 0 0 0 1 2 2 2
  line L155 (-23.5857, -6.7381) -> (-24.2788, -5.7489)
  spline S152 degree 2 poles (-24.2143, -3.1953) (-24.1648, -3.226) (-23.9914, -3.3269) (-23.9295, -3.382) knots 0 0 0 1 2 2 2
  spline S153 degree 2 poles (-23.9295, -3.382) (-23.8415, -3.4559) (-23.7181, -3.6114) (-23.6539, -3.7719) knots 0 0 0 1 2 2 2
  spline S154 degree 2 poles (-23.6539, -3.7719) (-23.6017, -3.9027) (-23.6059, -4.1783) (-23.6596, -4.3035) knots 0 0 0 1 2 2 2
  spline S155 degree 2 poles (-23.6596, -4.3035) (-23.7128, -4.4232) (-23.9284, -4.6291) (-24.0706, -4.686) knots 0 0 0 1 2 2 2
  spline S156 degree 2 poles (-24.0706, -4.686) (-24.2908, -4.774) (-24.677, -4.7129) (-24.8471, -4.5468) knots 0 0 0 1 2 2 2
  spline S157 degree 2 poles (-24.8471, -4.5468) (-25.0012, -4.4009) (-25.2575, -3.9395) (-25.3863, -3.6638) knots 0 0 0 1 2 2 2
  line L156 (-25.3863, -3.6638) -> (-25.4551, -3.6913)
  spline S158 degree 2 poles (-25.4551, -3.6913) (-25.579, -3.7408) (-25.7024, -3.8779) (-25.7185, -3.9641) knots 0 0 0 1 2 2 2
  spline S159 degree 2 poles (-25.7185, -3.9641) (-25.7345, -4.0503) (-25.6832, -4.2586) (-25.641, -4.3641) knots 0 0 0 1 2 2 2
  spline S160 degree 2 poles (-25.641, -4.3641) (-25.5915, -4.4879) (-25.3843, -4.7935) (-25.2462, -4.9325) knots 0 0 0 1 2 2 2
  line L157 (-25.2462, -4.9325) -> (-25.238, -4.9531)
  line L158 (-25.238, -4.9531) -> (-25.6027, -5.0989)
  spline S161 degree 2 poles (-25.6027, -5.0989) (-25.6696, -5.0113) (-25.886, -4.6695) (-25.9585, -4.4883) knots 0 0 0 1 2 2 2
  spline S162 degree 2 poles (-25.9585, -4.4883) (-26.0465, -4.2681) (-26.0978, -3.9402) (-26.056, -3.7852) knots 0 0 0 1 2 2 2
  spline S163 degree 2 poles (-26.056, -3.7852) (-26.0156, -3.6334) (-25.7839, -3.4077) (-25.5844, -3.328) knots 0 0 0 1 2 2 2
  line L159 (-25.5844, -3.328) -> (-24.1326, -2.7476)
  line L160 (-24.1326, -2.7476) -> (-23.9895, -3.1054)
  line L161 (-23.9895, -3.1054) -> (-24.2143, -3.1953)
  line L162 (-24.5125, -3.3144) -> (-25.1019, -3.5501)
  spline S164 degree 2 poles (-25.1019, -3.5501) (-25.0391, -3.6739) (-24.8452, -4.046) (-24.7599, -4.1528) knots 0 0 0 1 2 2 2
  spline S165 degree 2 poles (-24.7599, -4.1528) (-24.6595, -4.2776) (-24.404, -4.391) (-24.2435, -4.3268) knots 0 0 0 1 2 2 2
  spline S166 degree 2 poles (-24.2435, -4.3268) (-24.06, -4.2534) (-23.9567, -3.9728) (-24.0356, -3.7755) knots 0 0 0 1 2 2 2
  spline S167 degree 2 poles (-24.0356, -3.7755) (-24.1025, -3.6081) (-24.357, -3.3906) (-24.5125, -3.3144) knots 0 0 0 1 2 2 2
  line L163 (-24.3232, -1.8346) -> (-24.2411, -2.2111)
  line L164 (-24.2411, -2.2111) -> (-27.352, -2.889)
  line L165 (-27.352, -2.889) -> (-27.434, -2.5125)
  line L166 (-27.434, -2.5125) -> (-24.3232, -1.8346)
  point P0 (0, 0)
  dimension "d12" = 19
  constraints: 1 centre point, 1 coincident, 1 other
  measures "d12" diameter of A1
extrude "Vysunutí2" add sketch "Náčrt3" against normal blind 0.1 contours L73 S71 S72 S73 L74 L75 L76 L77 L78 S74 S75 S76 S77 S78 L79 L80 L70 S67 S68 S69 S70 L71 L72 | L108 L109 L110 L107 | L40 L41 L42 L43 L44 L45 S37 L46 L47 L48 L49 | S88 S89 S90 S91 L96 S92 S93 S94 L97 L98 S95 S96 S97 L99 L100 L101 S86 S87 A1 | A1 S87 S88 | S52 S53 A1 | A1 S53 S54 S55 S56 L63 S57 S58 S59 L64 L65 S60 S61 S62 L66 L67 L68 S51 S52 | S102 S103 S104 S105 S106 L103 L104 S107 S108 S109 S110 S111 L105 L106 S112 S113 A1 | A1 S113 S102 | S46 S38 A1 | A1 S38 S39 S40 S41 L58 L59 S42 S43 S44 L60 L61 S45 S46 | S122 L123 S123 S124 S125 S126 S127 L124 L125 L126 S128 A1 | A1 S128 S129 L127 L128 S119 S120 S121 S122 | S24 S25 A1 | A1 S25 S26 S27 S24 | S139 S140 S141 S142 L151 L152 S143 S144 S145 L153 L154 S146 S147 A1 | A1 S147 S139 | S19 S11 A1 | A1 S11 S12 S13 S14 L17 L18 S15 S16 S17 L19 L20 S18 S19 | S154 S155 S156 S157 L156 S158 S159 S160 L157 L158 S161 S162 S163 L159 L160 L161 S152 S153 A1 | A1 S153 S154 | S1 S2 A1 | A1 S2 S3 S4 S5 S6 L13 L14 L15 L11 L12 S0 S1 | L164 L165 L166 A1 | L0 L1 L2 L3 L4 L5 L6 L7 | L22 L23 S32 S33 S34 L24 L25 L26 L27 L28 S35 S36 L29 | L30 L31 L32 L33 L34 L35 L36 L37 L38 L39 | L50 L51 L52 L53 L54 L55 L56 L57 | L81 L82 L83 L84 | L85 L86 L87 L88 L89 L90 L91 S79 S80 S81 L92 | L111 L112 L113 L114 | L115 L116 S114 S115 S116 L117 L118 L119 L120 L121 S117 S118 L122 | L130 L131 L132 L133 L134 L135 L136 L137 L138 L139 L140 L141 L142 | L143 L144 S134 S135 S136 L145 L146 L147 L148 L149 S137 S138 L150
